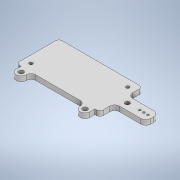
# Autodesk Inventor part: Part6
Saved by Autodesk Inventor 2021 (Build 250183000, 183)
## iProperties
Created: 2021-10-11
Part Number: Part6
Material: Generic
Document SubType Name: Modeling
Designer: Route
Density: 1 g/cm^3
Appearance: Default
Author: Route
Autodesk Inventor part; units mm, degrees
ref_plane "YZ Plane" through (0, 0, 0) normal (1, 0, 0) x (0, 1, 0)
ref_plane "XZ Plane" through (0, 0, 0) normal (0, 1, 0) x (-1, 0, 0)
ref_plane "XY Plane" through (0, 0, 0) normal (0, 0, 1) x (1, 0, 0)
sketch "Sketch1" plane through (0, 0, 0) normal (0, 1, 0) x (-1, 0, 0)
  circle A0 centre (25.2, -7) radius 1.35
  circle A1 centre (17.7, -7) radius 0.65
  circle A2 centre (15.2, -7) radius 0.65
  circle A3 centre (12.7, -7) radius 0.65
  line L0 (10, -7) -> (10, -8)
  line L1 (13, -11) -> (26, -11)
  line L2 (26, -3) -> (13, -3)
  line L3 (10, -6) -> (10, -7)
  arc A4 (13, -3) -> (10, -6) centre (13, -6) ccw
  arc A5 (10, -8) -> (13, -11) centre (13, -8) ccw
  line L4 (29, -14) -> (29, -18)
  line L5 (31, -20) -> (78, -20)
  line L6 (80, -18) -> (80, 4)
  line L7 (78, 6) -> (31, 6)
  line L8 (29, 4) -> (29, 0)
  arc A6 (26, -3) -> (29, 0) centre (26, 0) ccw
  arc A7 (29, -14) -> (26, -11) centre (26, -14) ccw
  arc A8 (31, 6) -> (29, 4) centre (31, 4) ccw
  arc A9 (80, 4) -> (78, 6) centre (78, 4) ccw
  arc A10 (78, -20) -> (80, -18) centre (78, -18) ccw
  arc A11 (29, -18) -> (31, -20) centre (31, -18) ccw
  point P0 (0, 0)
  point P1 (10, -3)
  point P2 (29, -7)
  point P3 (29, -20)
  point P4 (80, -20)
  point P5 (80, 6)
  point P6 (29, 6)
  dimension "d0" = 2.7
  dimension "d1" = 1.3
  dimension "d2" = 1.3
  dimension "d3" = 1.3
  dimension "d4" = 3
  dimension "d5" = 13
  dimension "d6" = 51
  dimension "d7" = 26
  dimension "d8" = 3
  dimension "d9" = 2
  constraints: 18 end point, 16 point on circle, 16 tangent, 14 point on line, 12 centre point, 5 equal radius, 4 perpendicular, 1 vertical
  measures "d0" diameter of A0
  measures "d1" diameter of A1
  measures "d2" diameter of A2
  measures "d3" diameter of A3
  measures "d4" radius of A4
  measures "d5" distance of point (29, -7) point (29, -20)
  measures "d6" distance of point (29, -20) point (80, -20)
  measures "d7" distance of point (80, -20) point (80, 6)
  measures "d8" radius of A6
  measures "d9" radius of A8
extrude "Extrusion1" add sketch "Sketch1" along normal blind 3
sketch "Sketch2" plane through (0, 3, 0) normal (0, 1, 0) x (1, 0, 0)
  line L0 (-77, 17) -> (-32, 17)
  line L1 (-32, 17) -> (-32, -3)
  line L2 (-32, -3) -> (-77, -3)
  line L3 (-77, -3) -> (-77, 17)
  line L4 (-78, 20) -> (-31, 20)
  line L5 (-29, 18) -> (-29, -4)
  line L6 (-41, -6) -> (-68, -6)
  line L7 (-80, -4) -> (-80, 18)
  arc A0 (-78, 20) -> (-80, 18) centre (-78, 18) ccw
  arc A1 (-29, 18) -> (-31, 20) centre (-31, 18) ccw
  arc A2 (-31, -6) -> (-29, -4) centre (-31, -4) ccw
  arc A3 (-80, -4) -> (-78, -6) centre (-78, -4) ccw
  line L8 (-77, -3) -> (-75.5, -3)
  line L9 (-75.5, -3) -> (-75.5, -1.5)
  circle A4 centre (-75.5, -1.5) radius 1
  line L10 (-32, 17) -> (-33.5, 17)
  line L11 (-33.5, 17) -> (-33.5, 15.5)
  circle A5 centre (-33.5, 15.5) radius 1
  line L12 (-49.42, 17) -> (-59.58, 17)
  line L13 (-59.58, 17) -> (-59.58, 14.46)
  line L14 (-59.58, 14.46) -> (-49.42, 14.46)
  line L15 (-49.42, 14.46) -> (-49.42, 17)
  line L16 (-78, -6) -> (-31, -6) projected
  line L17 (-77, -6) -> (-71, -6)
  line L18 (-71, -9) -> (-71, -9)
  line L19 (-74, -12) -> (-74, -12)
  line L20 (-77, -9) -> (-77, -6)
  line L21 (-32, -6) -> (-38, -6)
  line L22 (-38, -9) -> (-38, -9)
  line L23 (-35, -12) -> (-35, -12)
  line L24 (-32, -9) -> (-32, -6)
  arc A6 (-77, -9) -> (-74, -12) centre (-74, -9) ccw
  arc A7 (-74, -12) -> (-71, -9) centre (-74, -9) ccw
  arc A8 (-68, -6) -> (-71, -9) centre (-68, -9) ccw
  arc A9 (-38, -9) -> (-41, -6) centre (-41, -9) ccw
  arc A10 (-38, -9) -> (-35, -12) centre (-35, -9) ccw
  arc A11 (-35, -12) -> (-32, -9) centre (-35, -9) ccw
  circle A12 centre (-74, -9) radius 1.5
  circle A13 centre (-35, -9) radius 1.5
  line L25 (-77, -6) -> (-68, -6)
  line L26 (-41, -6) -> (-32, -6)
  point P0 (0, 0)
  point P1 (-38, -12)
  dimension "d12" = 45
  dimension "d13" = 20
  dimension "d14" = 2
  dimension "d15" = 1.5
  dimension "d16" = 1.5
  dimension "d17" = 2
  dimension "d18" = 1.5
  dimension "d19" = 1.5
  dimension "d20" = 2
  dimension "d22" = 10.16
  dimension "d23" = 2.54
  dimension "d24" = 3
  dimension "d25" = 3
  dimension "d26" = 3
  constraints: 52 end point, 20 point on circle, 20 tangent, 14 centre point, 13 point on line, 9 perpendicular, 8 equal radius, 8 parallel, 4 coincident, 4 horizontal, 2 collinear
  measures "d12" distance of L1.end L2.end
  measures "d13" distance of L0.end L1.end
  measures "d14" radius of A0
  measures "d15" distance of L2.end L8.end
  measures "d16" distance of L8.end L9.end
  measures "d17" diameter of A4
  measures "d18" distance of L0.end L10.end
  measures "d19" distance of L10.end L11.end
  measures "d20" diameter of A5
  measures "d22" distance of L12.start L12.end
  measures "d23" distance of L12.end L13.end
  measures "d24" radius of A6
  measures "d25" diameter of A12
  measures "d26" diameter of A13
extrude "Extrusion2" add sketch "Sketch2" against normal blind 3 contours L16 A8 A7 A6 L20 | L24 A11 A10 A9 L16
sketch "Sketch3" plane through (0, 3, 0) normal (0, 1, 0) x (1, 0, 0)
  line L0 (-77, 17) -> (-32, 17)
  line L1 (-32, 17) -> (-32, -3)
  line L2 (-32, -3) -> (-77, -3)
  line L3 (-77, -3) -> (-77, 17)
  line L4 (-78, 20) -> (-31, 20)
  line L5 (-29, 18) -> (-29, -4)
  line L6 (-41, -6) -> (-68, -6)
  line L7 (-80, -4) -> (-80, 18)
  arc A0 (-78, 20) -> (-80, 18) centre (-78, 18) ccw
  arc A1 (-29, 18) -> (-31, 20) centre (-31, 18) ccw
  arc A2 (-31, -6) -> (-29, -4) centre (-31, -4) ccw
  arc A3 (-80, -4) -> (-78, -6) centre (-78, -4) ccw
  line L8 (-77, -3) -> (-75.5, -3)
  line L9 (-75.5, -3) -> (-75.5, -1.5)
  circle A4 centre (-75.5, -1.5) radius 1
  line L10 (-32, 17) -> (-33.5, 17)
  line L11 (-33.5, 17) -> (-33.5, 15.5)
  circle A5 centre (-33.5, 15.5) radius 1
  line L12 (-49.42, 17) -> (-59.58, 17)
  line L13 (-59.58, 17) -> (-59.58, 14.46)
  line L14 (-59.58, 14.46) -> (-49.42, 14.46)
  line L15 (-49.42, 14.46) -> (-49.42, 17)
  line L16 (-78, -6) -> (-31, -6)
  line L17 (-77, -6) -> (-71, -6)
  line L18 (-71, -9) -> (-71, -9)
  line L19 (-74, -12) -> (-74, -12)
  line L20 (-77, -9) -> (-77, -6)
  line L21 (-32, -6) -> (-38, -6)
  line L22 (-38, -9) -> (-38, -9)
  line L23 (-35, -12) -> (-35, -12)
  line L24 (-32, -9) -> (-32, -6)
  arc A6 (-77, -9) -> (-74, -12) centre (-74, -9) ccw
  arc A7 (-74, -12) -> (-71, -9) centre (-74, -9) ccw
  arc A8 (-68, -6) -> (-71, -9) centre (-68, -9) ccw
  arc A9 (-38, -9) -> (-41, -6) centre (-41, -9) ccw
  arc A10 (-38, -9) -> (-35, -12) centre (-35, -9) ccw
  arc A11 (-35, -12) -> (-32, -9) centre (-35, -9) ccw
  circle A12 centre (-74, -9) radius 1.5
  circle A13 centre (-35, -9) radius 1.5
  line L25 (-77, -6) -> (-68, -6)
  line L26 (-41, -6) -> (-32, -6)
  point P0 (0, 0)
  point P1 (-38, -12)
  dimension "d29" = 45
  dimension "d30" = 20
  dimension "d31" = 2
  dimension "d32" = 1.5
  dimension "d33" = 1.5
  dimension "d34" = 2
  dimension "d35" = 1.5
  dimension "d36" = 1.5
  dimension "d37" = 2
  dimension "d38" = 10.16
  dimension "d39" = 2.54
  dimension "d40" = 3
  dimension "d41" = 3
  dimension "d42" = 3
  constraints: 54 end point, 20 point on circle, 20 tangent, 14 centre point, 13 point on line, 9 perpendicular, 8 equal radius, 8 parallel, 4 coincident, 4 horizontal, 2 collinear
  measures "d29" distance of L2.start L2.end
  measures "d30" distance of L0.end L2.start
  measures "d31" radius of A0
  measures "d32" distance of L2.end L9.start
  measures "d33" distance of L9.start L9.end
  measures "d34" diameter of A4
  measures "d35" distance of L0.end L11.start
  measures "d36" distance of L11.start L11.end
  measures "d37" diameter of A5
  measures "d38" distance of L12.start L13.start
  measures "d39" distance of L13.start L13.end
  measures "d40" radius of A6
  measures "d41" diameter of A12
  measures "d42" diameter of A13
extrude "Extrusion3" cut sketch "Sketch3" against normal blind 3 contours A4 | A5
body "Solid1"
